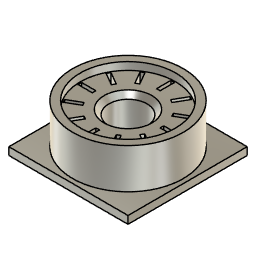
T_Nut_Mounting_Positive (Autodesk Fusion 360 design; units mm, degrees)
Autodesk Fusion 360 part; units mm, degrees
sketch "Sketch1" plane through (0, 0, 0) normal (0, 1, 0) x (1, 0, 0)
  line L0 (0, 0) -> (11.6, 0)
  line L1 (11.6, 0) -> (11.6, -10)
  line L2 (11.6, -10) -> (0, -10)
  line L3 (0, -10) -> (0, 0)
  line L4 (10, -10) -> (0, -10)
  line L5 (0, -10) -> (0, -8.4)
  line L6 (0, -8.4) -> (10, -8.4)
  line L7 (10, -8.4) -> (10, -10)
  line L8 (4, -8.4) -> (0, -8.4)
  line L9 (0, -8.4) -> (0, 0)
  line L10 (0, 0) -> (4, 0)
  line L11 (4, 0) -> (4, -8.4)
  line L12 (4, -7.4) -> (5, -8.4)
  dimension "d1" = 1.6
  dimension "d2" = 1.6
  dimension "d3" = 10
  dimension "d5" = 8.4
  dimension "d6" = 4
  dimension "d8" = 1
  dimension "d9" = 45
  constraint horizontal L0
  constraint vertical L1
  constraint horizontal L2
  constraint vertical L3
  constraint coincident L0.start L3.end
  constraint horizontal L4
  constraint vertical L5
  constraint horizontal L6
  constraint vertical L7
  constraint coincident L3 L5.end
  constraint coincident L2 L4.start
  constraint horizontal L8
  constraint vertical L9
  constraint horizontal L10
  constraint vertical L11
  constraint coincident L6 L8.start
  constraint coincident L11 L12.start
  constraint coincident L6 L12.end
  measures "d1" distance of L4.start L6.end
  measures "d2" distance of L1.end L4.start
  measures "d3" distance of L2.end L4.start
  measures "d5" distance of L8.start L10.end
  measures "d6" distance of L9 L11
  measures "d8" vertical distance of L12.start L12.end
  measures "d9" angle of L11 L12
revolve "Revolve1" add sketch "Sketch1" angle 360 about axis through (0, 0, 10) along (0, 0, -1) contours L0 L1 L2 L6 L7 L11 L12
sketch "Sketch2" plane through (0, 0, 0) normal (0, 0, -1) x (1, 0, 0)
  circle A0 centre (0, 0) radius 4
  circle A1 centre (0, 0) radius 11.6
  line L0 (-12.5, 12.5) -> (12.5, 12.5)
  line L1 (12.5, 12.5) -> (12.5, -12.5)
  line L2 (12.5, -12.5) -> (-12.5, -12.5)
  line L3 (-12.5, -12.5) -> (-12.5, 12.5)
  line L4 (-12.5, 12.5) -> (12.5, -12.5) construction
  line L5 (12.5, 12.5) -> (-12.5, -12.5) construction
  dimension "d10" = 25
  constraint horizontal L0
  constraint perpendicular L0 L1
  constraint parallel L0 L2
  constraint parallel L1 L3
  constraint coincident L4 A0.centre
  constraint coincident L5 A0.centre
  constraint coincident A0.centre A1.centre
  constraint equal L0 L3
  measures "d10" distance of L0.start L0.end
extrude "Extrude1" add sketch "Sketch2" against normal blind 1.6 contours L0 L1 L2 L3
sketch "Sketch3" plane through (0, 0, 8.4) normal (0, 0, 1) x (-1, 0, 0)
  circle A0 centre (0, 0) radius 10
  circle A1 centre (0, 0) radius 5
  line L0 (9.75, 0) -> (6.75, 0)
  line L1 (6.75, 0) -> (6.75, 0.75)
  line L2 (6.75, 0.75) -> (9.75, 0.75)
  line L3 (9.75, 0.75) -> (9.75, 0)
  dimension "d13" = 3
  dimension "d14" = 6.75
  dimension "d15" = 0.75
  constraint horizontal L0
  constraint vertical L1
  constraint horizontal L2
  constraint vertical L3
  constraint horizontal A0.centre L0.end
  measures "d13" distance of L0.start L0.end
  measures "d14" distance of A0.centre L0.end
  measures "d15" distance of L0.start L2.end
extrude "Extrude2" cut sketch "Sketch3" against normal blind 4.4 contours L0 L1 L2 L3
pattern_circular "C-Pattern1" count 12 over 360 about axis through (0, 0, 0) along (0, 0, 1) of "Extrude2"
